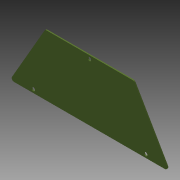
# Autodesk Inventor part: Veroboard
Saved by Autodesk Inventor 2015 (Build 190159000, 159)
## iProperties
Created: 2016-02-26
Part Number: Veroboard
Material: Generic
Document SubType Name: Modeling
Designer: James Yelland
Density: 1 g/cm^3
Appearance: Default
Author: James Yelland
Autodesk Inventor part; units mm, degrees
ref_plane "YZ Plane" through (0, 0, 0) normal (1, 0, 0) x (0, 1, 0)
ref_plane "XZ Plane" through (0, 0, 0) normal (0, 1, 0) x (-1, 0, 0)
ref_plane "XY Plane" through (0, 0, 0) normal (0, 0, 1) x (1, 0, 0)
sketch "Sketch1" plane through (0, 0, 0) normal (0, 1, 0) x (-1, 0, 0)
  circle A0 centre (-37, 5.818) radius 1.6079
  circle A1 centre (13.7917, 54.8205) radius 1.6079
  line L0 (13.7917, 57.8205) -> (-25.0536, 57.8205)
  line L1 (-26.7857, 56.8205) -> (-56.232, 5.818)
  line L2 (64.5833, 2.818) -> (-37, 2.818)
  line L3 (-54.5, 2.818) -> (-37, 2.818)
  line L4 (13.7917, 57.8205) -> (52.637, 57.8205)
  line L5 (54.369, 56.8205) -> (83.8153, 5.818)
  line L6 (82.0833, 2.818) -> (64.5833, 2.818)
  circle A2 centre (64.5833, 5.818) radius 1.6079
  arc A3 (82.0833, 2.818) -> (83.8153, 5.818) centre (82.0833, 4.818) ccw
  arc A4 (-56.232, 5.818) -> (-54.5, 2.818) centre (-54.5, 4.818) ccw
  arc A5 (-25.0536, 57.8205) -> (-26.7857, 56.8205) centre (-25.0536, 55.8205) ccw
  arc A6 (54.369, 56.8205) -> (52.637, 57.8205) centre (52.637, 55.8205) ccw
  dimension "d13" = 2
  dimension "d14" = 2
  constraints: 14 end point, 8 point on circle, 8 tangent, 7 centre point, 2 equal radius, 1 horizontal
  measures "d13" radius of A3
  measures "d14" radius of A6
extrude "Extrusion1" add sketch "Sketch1" along normal blind 1
body "Solid1"
